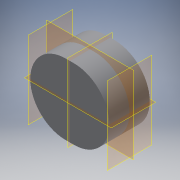
# Autodesk Inventor part: TAZ 6 Convex Model
Saved by Autodesk Inventor 2019 (Build 230136000, 136)
## iProperties
Created: 2021-02-10
Part Number: TAZ 6 Convex Model
Material: Generic
Document SubType Name: Modeling
Designer: Eric
Density: 1 g/cm^3
Appearance: Default
Author: Eric
Autodesk Inventor part; units mm, degrees
ref_plane "XZ Plane" through (0, 0, 0) normal (0, 1, 0) x (-1, 0, 0)
ref_plane "XY Plane" through (0, 0, 0) normal (0, 0, 1) x (1, 0, 0)
sketch "Sketch7" plane through (0, 0, 0) normal (0, 0, 1) x (1, 0, 0)
  line L0 (484, 161.1598) -> (484, 161.1598)
  line L1 (484, 153.6598) -> (484, 153.6598)
  line L2 (484, 161.1598) -> (484, 161.1598)
  line L3 (484, 153.6598) -> (484, 153.6598)
  line L4 (15, 0) -> (-15, 0) construction
  line L5 (15, 125) -> (-15, 125)
  line L6 (-15, -125) -> (15, -125)
  arc A0 (15, -125) -> (15, 125) centre (15, 0) ccw
  arc A1 (-15, 125) -> (-15, -125) centre (-15, 0) ccw
  point P0 (0, 0)
  point P1 (0, 0)
  dimension "d25" = 30
  dimension "d26" = 250
  constraints: 16 end point, 4 point on circle, 4 tangent, 2 centre point, 1 coincident, 1 horizontal, 1 midpoint, 1 parallel
  measures "d25" distance of L4.start L4.end
  measures "d26" diameter of A1
extrude "Extrusion5" add sketch "Sketch7" along normal blind 143
ref_plane "Work Plane11" through (-15, 0, 0) normal (0, 1, 0) x (1, 0, 0)
ref_plane "Work Plane12" through (0, 0, 71.5) normal (0, 0, 1) x (1, 0, 0)
ref_plane "Work Plane15" through (0, 0, 0) normal (1, 0, 0) x (0, 1, 0)
ref_plane "Work Plane13" through (140, 0, 0) normal (1, 0, 0) x (0, 1, 0)
ref_plane "Work Plane14" through (-140, 0, 0) normal (1, 0, 0) x (0, 1, 0)
body "Solid1"
body "Solid5"
